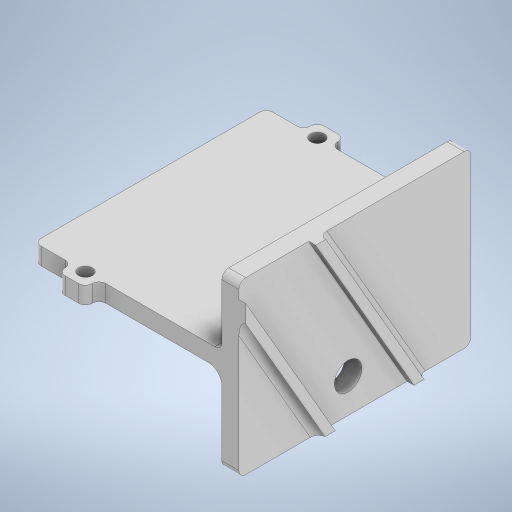
# Autodesk Inventor part: Part
Saved by Autodesk Inventor 2023 (Build 270158000, 158)
## iProperties
Created: 2024-08-18
Part Number: Part
Material: Generic
Document SubType Name: Modeling
Designer: Admins
Density: 1 g/cm^3
Appearance: Default
Author: Admins
Autodesk Inventor part; units mm, degrees
ref_plane "YZ Plane" through (0, 0, 0) normal (1, 0, 0) x (0, 1, 0)
ref_plane "XZ Plane" through (0, 0, 0) normal (0, 1, 0) x (-1, 0, 0)
ref_plane "XY Plane" through (0, 0, 0) normal (0, 0, 1) x (1, 0, 0)
sketch "Sketch1" plane through (0, 0, 0) normal (0, 1, 0) x (-1, 0, 0)
  point P0 (0, 0)
sketch "Sketch2" plane through (0, 0, 0) normal (0, 1, 0) x (-1, 0, 0)
  line L0 (-10, 34) -> (10, 34)
  line L1 (10, 34) -> (10, -34)
  line L2 (10, -34) -> (-10, -34)
  line L3 (-10, -34) -> (-10, 34)
  line L4 (-10, 34) -> (10, -34) construction
  line L5 (10, 34) -> (-10, -34) construction
  line L6 (-10, 34) -> (-25, 34)
  line L7 (-25, 34) -> (-25, -34)
  line L8 (-25, -34) -> (-10, -34)
  line L9 (-10, -34) -> (-10, 34)
  line L10 (-10, 34) -> (30, 34)
  line L11 (30, 34) -> (30, -34)
  line L12 (30, -34) -> (-10, -34)
  line L13 (-10, -34) -> (-10, 34)
  line L14 (-10, -34) -> (-14, -34)
  line L15 (-14, -34) -> (-6, -34)
  line L16 (-6, -34) -> (-14, -34)
  line L17 (-10, 34) -> (-14, 34)
  line L18 (-14, 34) -> (-6, 34)
  line L19 (-14, 34) -> (-6, 34)
  line L20 (30, 34) -> (15, 34)
  line L21 (15, 34) -> (15, -34)
  line L22 (15, -34) -> (30, -34)
  line L23 (30, -34) -> (30, 34)
  circle A0 centre (15, -34) radius 2
  circle A1 centre (15, 34) radius 2
  line L24 (15, 34) -> (19, 34)
  line L25 (19, 34) -> (11, 34)
  line L26 (11, 34) -> (11, 38)
  line L27 (11, 38) -> (19, 38)
  line L28 (19, 38) -> (19, 34)
  line L29 (15, -34) -> (19, -34)
  line L30 (19, -34) -> (11, -34)
  line L31 (11, -34) -> (11, -38)
  line L32 (11, -38) -> (19, -38)
  line L33 (19, -38) -> (19, -34)
  point P0 (0, 0)
  point P1 (10, 34)
  point P2 (13, 34)
  point P3 (17, 34)
  point P4 (17, -34)
  point P5 (13, -34)
  point P6 (10, 34)
  dimension "d0" = 20
  dimension "d1" = 68
  dimension "d4" = 15
  dimension "d5" = 40
  dimension "d10" = 4
  dimension "d11" = 8
  dimension "d42" = 15
  dimension "d43" = 4
  dimension "d44" = 4
  dimension "d45" = 4
  dimension "d46" = 8
  dimension "d47" = 4
  dimension "d48" = 8
  dimension "d49" = 4
  constraints: 68 end point, 12 parallel, 8 horizontal, 8 point on line, 6 perpendicular, 3 coincident, 2 centre point, 2 midpoint
  measures "d0" distance of L1.end L2.end
  measures "d1" distance of L0.end L1.end
  measures "d4" distance of L8.end L7.end
  measures "d5" distance of L11.end L12.end
  measures "d10" distance of L6.start L17.end
  measures "d11" distance of L17.end L18.end
  measures "d42" distance of L22.end L21.end
  measures "d43" diameter of A0
  measures "d44" diameter of A1
  measures "d45" distance of L24.start L24.end
  measures "d46" distance of L26.end L27.end
  measures "d47" distance of L29.start L29.end
  measures "d48" distance of L32.end L31.end
  measures "d49" distance of L31.end L30.end
sketch "Sketch3" plane through (0, 0, 0) normal (0, 1, 0) x (-1, 0, 0)
  point P0 (0, 0)
extrude "Extrusion1" add sketch "Sketch2" along normal blind 5 contours L0 L1 L2 L3 | L3 L8 L7 L6 | L10 A1 L21 A0 L12 L1 | L10 L21 A1 | A0 L21 L12 | L10 A1 L21 | L10 L11 L12 A0 L21 A1 | L21 A0 L12
sketch "Sketch4" plane through (0, 0, 0) normal (0, -1, 0) x (1, 0, 0)
  point P0 (0, 0)
sketch "Sketch5" plane through (-30, 0, -34) normal (-1, 0, 0) x (0, 0, 1)
  point P0 (34, 0)
sketch "Sketch6" plane through (25, 0, 34) normal (1, 0, 0) x (0, 0, -1)
  line L0 (0, -25) -> (68, -25)
  line L1 (68, -25) -> (68, 25)
  line L2 (68, 25) -> (0, 25)
  line L3 (0, 25) -> (0, -25)
  line L4 (0, -25) -> (68, 25) construction
  line L5 (68, -25) -> (0, 25) construction
  point P0 (34, 0)
  dimension "d16" = 50
  dimension "d41" = 68
  constraints: 12 end point, 2 midpoint, 2 parallel, 1 horizontal, 1 perpendicular
  measures "d16" distance of L1.end L0.end
  measures "d41" distance of L0.start L0.end
extrude "Extrusion2" add sketch "Sketch6" along normal blind 5
fillet "Face Fillet1" radius 2 1 edges at (25, 5, 0)
sketch "Sketch7" plane through (30, 0, 34) normal (1, 0, 0) x (0, 0, -1)
  line L0 (68, -25) -> (68, 0) projected
  line L1 (0, 25) -> (68, 25)
  line L2 (68, 25) -> (68, -15)
  line L3 (68, -15) -> (0, -15)
  line L4 (0, -15) -> (0, 25)
  line L5 (0, -15) -> (32, -15)
  circle A0 centre (32, -15) radius 4
  point P0 (34, 0)
  dimension "d20" = 40
  dimension "d21" = 32
  dimension "d22" = 8
  constraints: 10 end point, 2 parallel, 2 point on line, 1 centre point, 1 coincident, 1 horizontal, 1 perpendicular
  measures "d20" distance of L1.end L2.end
  measures "d21" distance of L3.end L5.end
  measures "d22" diameter of A0
extrude "Extrusion3" cut sketch "Sketch7" against normal through all contours A0 L3 | L3 A0
sketch "Sketch8" plane through (30, 0, 34) normal (1, 0, 0) x (0, 0, -1)
  line L0 (68, -25) -> (68, 0) projected
  line L1 (0, 25) -> (68, 25)
  line L2 (68, 25) -> (68, -15)
  line L3 (68, -15) -> (0, -15)
  line L4 (0, -15) -> (0, 25)
  line L5 (0, -15) -> (34, -15)
  circle A0 centre (32, -15) radius 4 projected
  line L6 (32, -15) -> (8.906, 25)
  line L7 (68, 25) -> (0, 25) projected
  line L8 (32, -15) -> (78.188, -15) construction
  line L9 (32, -15) -> (37.7735, -25)
  line L10 (0, -25) -> (68, -25) projected
  line L11 (16, 12.7128) -> (24.6603, 17.7128)
  line L12 (24.6603, 17.7128) -> (7.3397, 7.7128)
  line L13 (7.3397, 7.7128) -> (26.2265, -25)
  line L14 (26.2265, -25) -> (0, 20.4256)
  line L15 (0, 25) -> (0, -25) projected
  line L16 (24.6603, 17.7128) -> (49.3205, -25)
  line L17 (24.6603, 17.7128) -> (20.453, 25)
  line L18 (20.453, 25) -> (23.453, 25)
  line L19 (23.453, 25) -> (52.3205, -25)
  line L20 (26.2265, -25) -> (23.2265, -25)
  line L21 (23.2265, -25) -> (0, 15.2295)
  point P0 (34, 0)
  point P1 (0, 7)
  point P2 (0, 20.4256)
  point P3 (23.453, 25)
  point P4 (20.453, 25)
  dimension "d25" = 40
  dimension "d26" = 120
  dimension "d27" = 10
  dimension "d28" = 20
  dimension "d29" = 3
  dimension "d30" = 3
  constraints: 36 end point, 15 point on line, 5 parallel, 3 perpendicular, 2 horizontal, 1 equal length, 1 midpoint
  measures "d25" distance of L1.end L2.end
  measures "d26" angle of L8 L6
  measures "d27" distance of L11.start L11.end
  measures "d28" distance of L11.end L12.end
  measures "d29" distance of L17.end L18.end
  measures "d30" distance of L13.end L20.end
extrude "Extrusion4" add sketch "Sketch8" along normal blind 2 contours L10 L16 L3 L19 | L3 L16 L17 L1 L19 | L10 L21 L3 L13 | L3 L21 L4 L14 L13
fillet "Face Fillet2" radius 4 1 edges at (25, 0, 0)
fillet "Face Fillet3" radius 2 1 edges at (30, 0, -3.8868)
fillet "Face Fillet4" radius 2 1 edges at (30, -4.8853, 22.3868)
fillet "Fillet1" radius 2 6 edges at (-30, 2.5, -34) (-30, 2.5, 34) (27.5, -25, 34) (27.5, -25, -34) (27.5, 25, -34) (27.5, 25, 34)
extrude "Extrusion5" add sketch "Sketch2" along normal blind 5 contours L26 L27 L28 L10 A1
extrude "Extrusion6" add sketch "Sketch2" along normal blind 5 contours L12 A0 L33 L32 L31
extrude "Extrusion7" cut sketch "Sketch2" along normal blind 5 contours A0 L21 L12 | L21 A0 L12
extrude "Extrusion8" cut sketch "Sketch2" along normal blind 5 contours L10 L21 A1 | L10 A1 L21
fillet "Fillet2" radius 2 4 edges at (-19, 2.5, 38) (-11, 2.5, 38) (-19, 2.5, -38) (-11, 2.5, -38)
fillet "Face Fillet9" radius 2 1 edges at (-19, 2.5, 34)
fillet "Face Fillet10" radius 2 1 edges at (-11, 2.5, 34)
fillet "Face Fillet11" radius 2 1 edges at (-19, 2.5, -34)
fillet "Face Fillet12" radius 2 1 edges at (-11, 2.5, -34)
body "Solid1"
